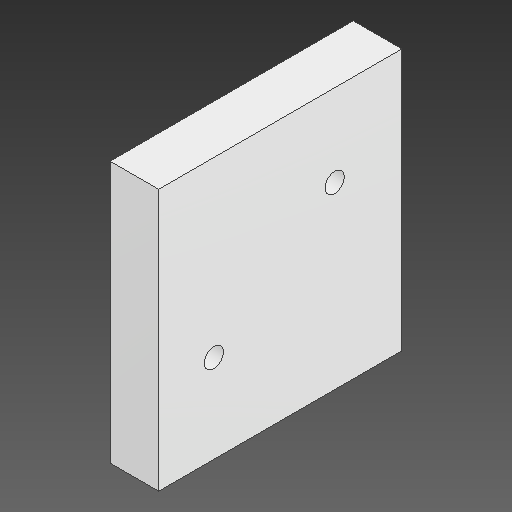
# Autodesk Inventor part: SmallFrontWallUHMW
Saved by Autodesk Inventor 2021 (Build 250183000, 183)
## iProperties
Created: 2021-03-10
Part Number: SmallFrontWallUHMW
Material: UHMW, White
Document SubType Name: Modeling
Designer: Dylan
Density: 0.94 g/cm^3
Appearance: Smooth - White
Mass: 410.165 g
Surface Area: 493.543 cm^2
Volume: 436.345 cm^3
Author: Dylan
Autodesk Inventor part; units mm, degrees
ref_plane "YZ Plane" through (0, 0, 0) normal (1, 0, 0) x (0, 1, 0)
ref_plane "XZ Plane" through (0, 0, 0) normal (0, 1, 0) x (-1, 0, 0)
ref_plane "XY Plane" through (0, 0, 0) normal (0, 0, 1) x (1, 0, 0)
sketch "Sketch1" plane through (0, 0, 0) normal (1, 0, 0) x (0, 1, 0)
  line L0 (31.75, -19.05) -> (168.275, -19.05)
  line L1 (168.275, -19.05) -> (168.275, -146.05)
  line L2 (168.275, -146.05) -> (31.75, -146.05)
  line L3 (31.75, -146.05) -> (31.75, -19.05)
  constraints: 8 end point, 2 coincident, 2 parallel, 1 horizontal, 1 perpendicular, 2 other
extrude "Extrusion1" add sketch "Sketch1" along normal blind 25.4
sketch "Sketch2" plane through (0, 0, 0) normal (-1, 0, 0) x (0, 0, 1)
  circle A0 centre (-110.9113, 125.4125) radius 5.0419 projected
  circle A1 centre (-47.8387, 77.7875) radius 5.0419 projected
  point P0 (0, 0)
hole "Hole1" at (0, 77.7875, -47.8387) at (0, 125.4125, -110.9113) direction (1, 0, 0) diameter 10.0838 end through all clearance for "Hex Head Bolt" size "3/8" standard "Ansi Unified Screw Threads"
body "Solid1"
